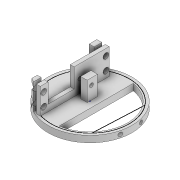
# Autodesk Inventor part: bae_nueva_piza
Saved by Autodesk Inventor 2021 (Build 250183000, 183)
## iProperties
Created: 2022-06-08
Part Number: bae_nueva_piza
Material: Genérico
Document SubType Name: Modeling
Designer: orgyn
Density: 1 g/cm^3
Appearance: Valor por defecto
Author: orgyn
Autodesk Inventor part; units mm, degrees
ref_plane "YZ Plane" through (0, 0, 0) normal (1, 0, 0) x (0, 1, 0)
ref_plane "XZ Plane" through (0, 0, 0) normal (0, 1, 0) x (-1, 0, 0)
ref_plane "XY Plane" through (0, 0, 0) normal (0, 0, 1) x (1, 0, 0)
sketch "Boceto1" plane through (0, 0, 0) normal (0, 1, 0) x (-1, 0, 0)
  circle A0 centre (0, 0) radius 32.5
  dimension "d8" = 65
  constraints: 1 centre point, 1 coincident
  measures "d8" diameter of A0
extrude "Extrusión1" add sketch "Boceto1" along normal blind 5
sketch "Boceto3" plane through (0, 5, 0) normal (0, 1, 0) x (1, 0, 0)
  line L0 (0, 0) -> (0, 7.5)
  line L1 (0, 7.5) -> (0, 24.1)
  line L2 (0, -29.34) -> (-9.2, -29.34)
  line L3 (0, 24.1) -> (0, -29.3)
  line L4 (-9.2, -29.34) -> (-9.2, 24.06)
  line L5 (-9.2, 24.06) -> (-12.2, 24.06)
  line L6 (-12.2, 24.06) -> (-12.2, -29.34)
  line L7 (-12.2, -29.34) -> (-9.2, -29.34)
  dimension "d9" = 7.5
  dimension "d10" = 16.6
  dimension "d11" = 53.44
  dimension "d12" = 9.2
  dimension "d14" = 53.4
  dimension "d15" = 53.4
  dimension "d16" = 3
  constraints: 16 end point, 3 perpendicular, 3 vertical, 2 point on line
  measures "d9" distance of L0.start L0.end
  measures "d10" distance of L0.end L1.end
  measures "d11" distance of L1.end L2.start
  measures "d12" distance of L2.start L2.end
  measures "d14" distance of L1.end L3.end
  measures "d15" distance of L2.end L4.end
  measures "d16" distance of L4.end L5.end
extrude "Extrusión2" add sketch "Boceto3" along normal blind 30
sketch "Boceto4" plane through (-9.2, 5, 29.34) normal (1, 0, 0) x (0, 0, -1)
  line L0 (0, 0) -> (53.4, 0) projected
  line L1 (0, 0) -> (0, 5.05)
  line L2 (0, 0) -> (0, 30) projected
  line L3 (0, 5.05) -> (53.4, 5.05)
  line L4 (53.4, 0) -> (53.4, 30) projected
  line L5 (0, 30) -> (0, 24.95)
  line L6 (0, 0) -> (0, 30) projected
  line L7 (0, 24.95) -> (53.4, 24.95)
  line L8 (0, 24.95) -> (2.6, 24.95)
  line L9 (2.6, 24.95) -> (2.6, 5.05)
  line L10 (53.4, 24.95) -> (50.8, 24.95)
  line L11 (50.8, 24.95) -> (50.8, 5.05)
  line L12 (2.6, 15) -> (2.6, 24.9)
  circle A0 centre (2.6, 24.95) radius 2.2
  circle A1 centre (2.6, 5.05) radius 2.2
  circle A2 centre (50.8, 24.95) radius 2.2
  circle A3 centre (50.8, 5.05) radius 2.2
  line L13 (0, 15) -> (53.4, 15)
  line L14 (0, 15) -> (16.6, 15)
  line L15 (16.6, 15) -> (16.6, 19.6462)
  line L16 (16.6, 15) -> (30.1, 15)
  circle A4 centre (30.1, 15) radius 1.5
  line L17 (26.2533, 15) -> (26.2533, 24.95)
  line L18 (26.2533, 15) -> (26.2533, 5.05)
  line L19 (53.4, 30) -> (0, 30) projected
  line L20 (0, 30) -> (6, 30)
  line L21 (0, 30) -> (53.4, 30) projected
  line L22 (6, 30) -> (6, 0)
  line L23 (53.4, 0) -> (0, 0) projected
  line L24 (53.4, 30) -> (47.4, 30)
  line L25 (47.4, 30) -> (47.4, 0)
  line L26 (2.6, 5.05) -> (2.6, 14.95)
  circle A5 centre (2.6, 14.95) radius 2.2
  circle A6 centre (50.8, 15) radius 2.2
  line L27 (2.6, 10) -> (50.8, 10)
  line L28 (30.1, 15) -> (30.1, 5.05)
  line L29 (0, 0) -> (0, 20)
  line L30 (0, 20) -> (53.4, 20)
  line L31 (28.6, 15) -> (33.0996, 15)
  point P0 (29.34, -5)
  point P1 (6, 5.05)
  point P2 (47.4, 24.95)
  point P3 (6, 20)
  point P4 (26.2533, 20)
  dimension "d31" = 3
  dimension "d19" = 5.05
  dimension "d20" = 5.05
  dimension "d22" = 2.6
  dimension "d23" = 2.6
  dimension "d24" = 9.9
  dimension "d25" = 4.4
  dimension "d26" = 4.4
  dimension "d27" = 4.4
  dimension "d28" = 4.4
  dimension "d29" = 16.6
  dimension "d30" = 13.5
  dimension "d32" = 6
  dimension "d33" = 6
  dimension "d41" = 9.9
  dimension "d42" = 4.4
  dimension "d43" = 4.4
  dimension "d44" = 20
  constraints: 50 end point, 27 point on line, 10 perpendicular, 6 centre point, 6 coincident, 5 midpoint, 1 horizontal alignment, 2 other
  measures "d19" distance of L0.start L1.end
  measures "d20" distance of L2.end L5.end
  measures "d22" distance of L5.end L8.end
  measures "d23" distance of L7.end L10.end
  measures "d24" distance of L12.start L12.end
  measures "d25" diameter of A0
  measures "d26" diameter of A1
  measures "d27" diameter of A2
  measures "d28" diameter of A3
  measures "d29" distance of L13.start L14.end
  measures "d30" distance of L14.end L16.end
  measures "d32" distance of L2.end L20.end
  measures "d33" distance of L4.end L24.end
  measures "d41" distance of L26.start L26.end
  measures "d42" diameter of A5
  measures "d43" diameter of A6
  measures "d44" distance of L0.start L29.end
extrude "Extrusión3" cut sketch "Boceto4" against normal blind 9.9 contours L22 L27 L18 L3 | A1 L9 L3 | L3 A1 | L3 L9 A1 | L22 L13 L18 L27 | L2 L7 A0 L9 L30 | A5 L9 L13 | L13 L9 A5 | A3 L11 L3 | L3 A3 | L22 L30 L17 L13 | L2 L19 L22 L7 A0 | L9 A0 L7 L22 L30 | L13 A5 L9 | L9 A5 L13 | L3 L11 A3 | L22 L7 L17 L30 | A0 L7 | L7 L9 A0 | L9 L7 A0 | L30 L11 A2 L7 L4 | A6 L11 L13 | L13 L11 A6 | A6 L11 L13 | L13 L11 A6 | L30 L17 L7 L25 | L25 L7 A2 L11 L30 | L22 L19 L25 L7 | L7 A2 L25 L19 L4 | A2 L11 L7 | L7 A2 | A2 L7 L11
sketch "Boceto5" plane through (0, 5, 0) normal (0, 1, 0) x (1, 0, 0)
  line L0 (-12.2, -29.34) -> (-12.2, 24.06) projected
  line L1 (-12.2, 24.06) -> (-14.8, 24.06)
  line L2 (-14.8, 24.06) -> (-14.8, -28.9346)
  circle A0 centre (0, 0) radius 32.5 projected
  line L3 (-12.2, -28.9346) -> (-14.8, -28.9346)
  line L4 (-14.8, 24.06) -> (-16.8, 24.06)
  line L5 (-16.8, 24.06) -> (-18.8, 24.06)
  line L6 (-18.8, 24.06) -> (-17.8, -28.9346)
  line L7 (-17.8, -28.9346) -> (-15.3324, -28.9346)
  line L8 (-18.8, 24.06) -> (-18.6868, 18.0611)
  line L9 (-18.6868, 18.0611) -> (-14.8, 18.0611)
  line L10 (-14.8, -28.9346) -> (-14.8, -22.9346)
  line L11 (-14.8, -22.9346) -> (-17.9121, -22.9933)
  point P0 (-17.8333, -27.1703)
  dimension "d36" = 2.6
  dimension "d37" = 2
  dimension "d38" = 2
  dimension "d45" = 6
  dimension "d46" = 6
  constraints: 22 end point, 8 point on line, 4 perpendicular, 1 horizontal, 2 other
  measures "d36" distance of L0.end L1.end
  measures "d37" distance of L1.end L4.end
  measures "d38" distance of L4.end L5.end
  measures "d45" distance of L5.end L8.end
  measures "d46" distance of L2.end L10.end
extrude "Extrusión4" add sketch "Boceto5" along normal blind 20 contours A0 L6 L11 L2 | L2 L9 L6 L5 L4
sketch "Boceto6" plane through (-18.6868, 5, -18.0611) normal (-0.9998, 0, 0.0189) x (0.0189, 0, 0.9998)
  ellipse E0 centre (-3.2193, 15) end of major axis (-3.2193, 12.8) minor radius 2.1996 projected
  circle A0 centre (-3.2193, 15) radius 2.2
  ellipse E1 centre (-3.2759, 5.05) end of major axis (-3.2759, 7.25) minor radius 2.1996 projected
  circle A1 centre (-3.2759, 5.05) radius 2.2
  ellipse E2 centre (44.9155, 14.95) end of major axis (44.9155, 17.15) minor radius 2.1996 projected
  circle A2 centre (44.9155, 14.95) radius 2.2
  ellipse E3 centre (44.9155, 5.05) end of major axis (44.9155, 7.25) minor radius 2.1996 projected
  circle A3 centre (44.9155, 5.05) radius 2.2
  point P0 (18.4104, -5)
  constraints: 4 centre point, 4 coincident, 8 other
extrude "Extrusión5" cut sketch "Boceto6" against normal blind 30
sketch "Boceto7" plane through (-9.2, 5, 29.34) normal (1, 0, 0) x (0, 0, -1)
  line L0 (2.1697, 20) -> (0.4054, 20) projected
  line L1 (26.2533, 20) -> (53.4, 20) projected
  line L2 (0, 0) -> (0, 20) projected
  line L3 (0, 20) -> (30.1, 20)
  line L4 (30.1, 20) -> (30.6, 20)
  line L5 (53.4, 20) -> (26.2533, 20) projected
  line L6 (30.6, 20) -> (30.6, 10)
  circle A0 centre (30.6, 10) radius 1.5
  point P0 (29.34, -5)
  dimension "d63" = 30.1
  dimension "d64" = 0.5
  dimension "d65" = 10
  dimension "d66" = 3
  constraints: 6 end point, 2 point on line, 1 centre point, 1 coincident, 1 perpendicular
  measures "d63" distance of L2.end L3.end
  measures "d64" distance of L3.end L4.end
  measures "d65" distance of L4.end L6.end
  measures "d66" diameter of A0
extrude "Extrusión6" cut sketch "Boceto7" against normal blind 5
sketch "Boceto8" plane through (0, 5, 0) normal (0, 1, 0) x (1, 0, 0)
  line L0 (-9.2, 24.06) -> (-9.2, -29.34) projected
  line L1 (-9.2, 24.06) -> (-5.2, 24.06)
  line L2 (-5.2, 24.06) -> (-5.2, 0)
  line L3 (-5.2, 0) -> (-0.2, 0)
  line L4 (-0.2, 0) -> (-0.2, 11.3407)
  line L5 (-9.2, -29.34) -> (-9.2, 0.76)
  line L6 (-9.6091, -29.34) -> (-9.2, -12.745)
  line L7 (-9.2, -12.745) -> (-9.2, -5.245)
  line L8 (-9.2, -5.245) -> (-9.2, 2.255)
  line L9 (-9.2, 2.255) -> (-9.2, 2.755)
  line L10 (-9.2, 2.76) -> (-9.2, -0.24) projected
  line L11 (-9.2, 2.76) -> (-0.2, 2.76)
  line L12 (-0.2, 0) -> (-0.2, 5.5)
  line L13 (-0.2, 0) -> (-0.2, 6)
  line L14 (-0.2, 6) -> (-5.2, 6)
  line L15 (-0.2, 0) -> (-0.2, -1)
  line L16 (-0.2, -1) -> (-5.2, -1)
  line L17 (-5.2, -1) -> (-5.2, -2)
  line L18 (-5.2, -2) -> (0, -2)
  line L19 (-5.2, 0) -> (-5.2, -1)
  line L20 (-0.2, -2) -> (-0.2, -1)
  point P0 (0, 0)
  dimension "d57" = 4
  dimension "d58" = 5
  dimension "d60" = 16.6
  dimension "d61" = 7.5
  dimension "d62" = 7.5
  dimension "d67" = 0.5
  dimension "d68" = 5.5
  dimension "d69" = 6
  dimension "d70" = 1
  dimension "d73" = 1
  constraints: 38 end point, 10 point on line, 6 perpendicular, 4 vertical, 2 horizontal
  measures "d57" distance of L0.start L1.end
  measures "d58" distance of L2.end L3.end
  measures "d60" distance of L6.start L6.end
  measures "d61" distance of L6.end L7.end
  measures "d62" distance of L7.end L8.end
  measures "d67" distance of L8.end L9.end
  measures "d68" distance of L3.end L12.end
  measures "d69" distance of L3.end L13.end
  measures "d70" distance of L3.end L15.end
  measures "d73" distance of L16.end L17.end
extrude "Extrusión7" add sketch "Boceto8" along normal blind 15 contours L11 L4 L3 L2 | L2 L14 L4 L11 | L3 L15 L16 L19 | L16 L20 L18 L17
sketch "Boceto10" plane through (-0.2, 5, 2) normal (1, 0, 0) x (0, 0, -1)
  circle A0 centre (3.26, 10) radius 1.5 projected
  circle A1 centre (3.26, 10) radius 1.5
  point P0 (2, -5)
  constraints: 1 centre point, 1 coincident
extrude "Extrusión8" cut sketch "Boceto10" against normal blind 20
sketch "Boceto11" plane through (0, 5, 0) normal (0, 1, 0) x (1, 0, 0)
  circle A0 centre (0, 0) radius 30.2549
  line L0 (22.0003, -20.7688) -> (23.8283, 18.6432)
  constraints: 2 end point, 2 point on circle, 1 centre point, 1 coincident
sketch "Boceto12" plane through (0, 0, 0) normal (0, -1, 0) x (1, 0, 0)
  line L0 (0, 0) -> (22.5, 0)
  line L1 (22.5, 0) -> (22.5, -22.5)
  line L2 (22.5, -22.5) -> (-22.5, -22.5)
  line L3 (-22.5, -22.5) -> (-22.5, 22.5)
  line L4 (-22.5, 22.5) -> (22.5, 22.5)
  line L5 (22.5, 22.5) -> (22.5, 0)
  circle A0 centre (0, 0) radius 29.116
  line L6 (4.8152, -22.5) -> (4.8152, 28.7151)
  line L7 (4.8152, -22.5) -> (4.8152, -28.7151)
  dimension "d76" = 22.5
  dimension "d77" = 22.5
  dimension "d78" = 45
  dimension "d79" = 45
  dimension "d80" = 45
  constraints: 16 end point, 4 perpendicular, 2 point on circle, 2 point on line, 2 vertical, 1 centre point, 1 coincident, 1 horizontal
  measures "d76" distance of L0.start L0.end
  measures "d77" distance of L0.end L1.end
  measures "d78" distance of L1.end L2.end
  measures "d79" distance of L2.end L3.end
  measures "d80" distance of L3.end L4.end
extrude "Extrusión9" cut sketch "Boceto12" against normal blind 20 contours L6 L4 A0 L5 L0 | L0 L1 A0 L2 L6 | L5 A0 L1 | L2 A0 L7 | L6 A0 L4 picked at (12.5348, -23.4523) picked at (12.5348, 23.4523)
sketch "Boceto13" plane through (4.8152, 0, 28.7151) normal (1, 0, 0) x (0, 0, -1)
  line L0 (57.4301, 0) -> (0, 0) projected
  line L1 (0, 0) -> (57.4301, 0)
  line L2 (28.7151, 0) -> (20.7151, 0)
  line L3 (20.7151, 0) -> (36.7151, 0)
  line L4 (20.7151, 0) -> (20.7151, 5)
  line L5 (0, 5) -> (57.4301, 5) projected
  line L6 (36.7151, 0) -> (36.7151, 5)
  circle A0 centre (20.7151, 2.5) radius 1.5
  circle A1 centre (36.7151, 2.5) radius 1.5
  dimension "d83" = 8
  dimension "d84" = 16
  dimension "d85" = 3
  dimension "d86" = 3
  constraints: 10 end point, 3 point on line, 2 centre point, 2 midpoint, 2 vertical, 1 collinear
  measures "d83" distance of L2.start L2.end
  measures "d84" distance of L2.end L3.end
  measures "d85" diameter of A0
  measures "d86" diameter of A1
extrude "Extrusión10" cut sketch "Boceto13" along normal blind 40 contours A1 L6 | L6 A1 | A0 L4 | L4 A0
equation "\"d34\" = d24"
